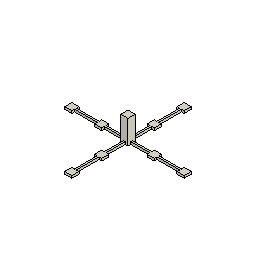
xy100mm (Autodesk Fusion 360 design; units mm, degrees)
Autodesk Fusion 360 part; units mm, degrees
sketch "Sketch1" plane through (0, 0, 0) normal (0, 0, 1) x (1, 0, 0)
  line L0 (0, 0) -> (0, 50) construction
  line L1 (3, 50) -> (-3, 50)
  line L2 (-3, 50) -> (-3, 44)
  line L3 (-3, 44) -> (3, 44)
  line L4 (3, 44) -> (3, 50)
  line L5 (3, 50) -> (-3, 44) construction
  line L6 (-3, 50) -> (3, 44) construction
  line L7 (3, 3) -> (-3, 3)
  line L8 (-3, 3) -> (-3, -3)
  line L9 (-3, -3) -> (3, -3)
  line L10 (3, -3) -> (3, 3)
  line L11 (3, 3) -> (-3, -3) construction
  line L12 (-3, 3) -> (3, -3) construction
  line L13 (0.75, 44) -> (0.75, 3)
  line L14 (-0.75, 44) -> (-0.75, 3)
  line L15 (-50, -3) -> (-44, -3)
  line L16 (-50, 3) -> (-50, -3)
  line L17 (-44, 3) -> (-50, 3)
  line L18 (-44, -3) -> (-44, 3)
  line L19 (-44, -0.75) -> (-3, -0.75)
  line L20 (-44, 0.75) -> (-3, 0.75)
  line L21 (3, -50) -> (3, -44)
  line L22 (-3, -50) -> (3, -50)
  line L23 (-3, -44) -> (-3, -50)
  line L24 (3, -44) -> (-3, -44)
  line L25 (0.75, -44) -> (0.75, -3)
  line L26 (-0.75, -44) -> (-0.75, -3)
  line L27 (50, 3) -> (44, 3)
  line L28 (50, -3) -> (50, 3)
  line L29 (44, -3) -> (50, -3)
  line L30 (44, 3) -> (44, -3)
  line L31 (44, 0.75) -> (3, 0.75)
  line L32 (44, -0.75) -> (3, -0.75)
  line L33 (3, 25) -> (-3, 25)
  line L34 (-3, 25) -> (-3, 19)
  line L35 (3, 19) -> (3, 25)
  line L36 (-3, 19) -> (3, 19)
  line L37 (-19, 3) -> (-25, 3)
  line L38 (-25, 3) -> (-25, -3)
  line L39 (-25, -3) -> (-19, -3)
  line L40 (-19, -3) -> (-19, 3)
  line L41 (-3, -19) -> (-3, -25)
  line L42 (-3, -25) -> (3, -25)
  line L43 (3, -25) -> (3, -19)
  line L44 (3, -19) -> (-3, -19)
  line L45 (19, -3) -> (25, -3)
  line L46 (25, -3) -> (25, 3)
  line L47 (25, 3) -> (19, 3)
  line L48 (19, 3) -> (19, -3)
  point P0 (0, 47)
  dimension "d1" = 50
  dimension "d2" = 6
  dimension "d3" = 6
  dimension "d4" = 6
  dimension "d5" = 6
  dimension "d6" = 1.5
  dimension "d8" = 360
  dimension "d13" = 6
  dimension "d14" = 6
  dimension "d15" = 25
  dimension "d17" = 360
  constraint coincident L0.start origin
  constraint vertical L0
  constraint horizontal L1
  constraint perpendicular L1 L2
  constraint parallel L1 L3
  constraint parallel L2 L4
  constraint coincident L5 P0
  constraint coincident L6 P0
  constraint coincident L0 P0
  constraint coincident L0.end L1
  constraint horizontal L7
  constraint perpendicular L7 L8
  constraint parallel L7 L9
  constraint parallel L8 L10
  constraint coincident L11 L0.start
  constraint coincident L12 L0.start
  constraint coincident L3 L13.start
  constraint coincident L7 L13.end
  constraint perpendicular L7 L13
  constraint symmetric L0 L13.start L14.start
  constraint symmetric L0 L13.end L14.end
  constraint horizontal L33
  constraint perpendicular L33 L34
  constraint parallel L33 L36
  constraint parallel L34 L35
  constraint symmetric L0 L34 L35
  measures "d1" distance of L0.start L0.end
  measures "d2" distance of L2.end L3.end
  measures "d3" distance of L1.end L2.end
  measures "d4" distance of L8.end L9.end
  measures "d5" distance of L7.end L8.end
  measures "d6" distance of L13 L14
  measures "d13" distance of L34.end L35.start
  measures "d14" distance of L33.end L34.end
  measures "d15" distance of L1 L33
extrude "Extrude1" add sketch "Sketch1" along normal blind 2
extrude "Extrude2" add sketch "Sketch1" along normal blind 20 contours L7 L8 L9 L10
